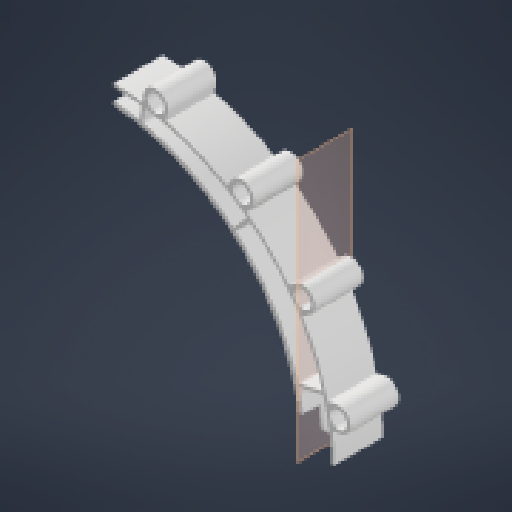
# Autodesk Inventor part: FilterSidewall
Saved by Autodesk Inventor 2026 (Build 300175050, 175E)
## iProperties
Created: 2026-05-05
Part Number: FilterSidewall
Material: Generic
Document SubType Name: Modeling
Designer: sniel
Density: 1 g/cm^3
Appearance: Default
Author: sniel
Autodesk Inventor part; units mm, degrees
ref_plane "YZ Plane" through (0, 0, 0) normal (1, 0, 0) x (0, 1, 0)
ref_plane "XZ Plane" through (0, 0, 0) normal (0, 1, 0) x (-1, 0, 0)
ref_plane "XY Plane" through (0, 0, 0) normal (0, 0, 1) x (1, 0, 0)
sketch "Sketch1" plane through (0, 0, 0) normal (0, 0, 1) x (1, 0, 0)
  circle A0 centre (-26.462672, 2.498755) radius 5.25
  circle A1 centre (-79.388016, -19.42364) radius 5.25
  circle A2 centre (-138.734281, -109.772854) radius 5.25
  circle A3 centre (-116.811886, -56.84751) radius 5.25
  line L0 (-70.374602, -19.468325) -> (-73.075282, -15.258264)
  arc A4 (-73.075282, -15.258264) -> (-85.476982, -23.686741) centre (-79.388065, -19.307803) ccw
  line L1 (-85.476982, -23.686741) -> (-82.556623, -27.747503)
  arc A5 (-82.556623, -27.747503) -> (-108.372236, -53.563116) centre (-0.000049, -136.119689) ccw
  line L2 (-108.372236, -53.563116) -> (-112.432997, -50.642756)
  arc A6 (-112.432997, -50.642756) -> (-120.861475, -63.044456) centre (-116.811935, -56.731673) ccw
  line L3 (-120.861475, -63.044456) -> (-116.651414, -65.745136)
  arc A7 (-116.651414, -65.745136) -> (-132.247344, -103.397042) centre (-0.000049, -136.119689) ccw
  line L4 (-132.247344, -103.397042) -> (-137.133976, -102.329748)
  arc A8 (-137.133976, -102.329748) -> (-139.943468, -117.058908) centre (-138.734331, -109.657017) ccw
  line L5 (-139.943468, -117.058908) -> (-135.00707, -117.865294)
  arc A9 (-135.00707, -117.865294) -> (-136.235526, -136.235526) centre (-0.000049, -136.119689) ccw
  line L6 (-136.235526, -136.235526) -> (-134.235526, -136.235526)
  arc A10 (0, -2) -> (-134.235526, -136.235526) centre (0, -136.235526) ccw
  line L7 (0, -2) -> (0, 0.115837)
  arc A11 (0, 0.115837) -> (-18.254444, -1.112668) centre (-0.000049, -136.119689) ccw
  line L8 (-18.254444, -1.112668) -> (-19.060831, 3.82373)
  arc A12 (-19.060831, 3.82373) -> (-33.78999, 1.014237) centre (-26.462721, 2.614592) ccw
  line L9 (-33.78999, 1.014237) -> (-32.722696, -3.872394)
  arc A13 (-32.722696, -3.872394) -> (-70.374602, -19.468325) centre (-0.000049, -136.119689) ccw
  circle A14 centre (138.734281, -109.772854) radius 5.25
  circle A15 centre (116.811886, -56.84751) radius 5.25
  circle A16 centre (26.462672, 2.498755) radius 5.25
  circle A17 centre (79.388016, -19.42364) radius 5.25
  line L10 (116.651364, -65.745136) -> (120.861425, -63.044456)
  arc A18 (120.861425, -63.044456) -> (112.432948, -50.642756) centre (116.811886, -56.731673) ccw
  line L11 (112.432948, -50.642756) -> (108.372186, -53.563116)
  arc A19 (108.372186, -53.563116) -> (82.556573, -27.747503) centre (0, -136.119689) ccw
  line L12 (82.556573, -27.747503) -> (85.476933, -23.686741)
  arc A20 (85.476933, -23.686741) -> (73.075233, -15.258264) centre (79.388016, -19.307803) ccw
  line L13 (73.075233, -15.258264) -> (70.374553, -19.468325)
  arc A21 (70.374553, -19.468325) -> (32.722647, -3.872394) centre (0, -136.119689) ccw
  line L14 (32.722647, -3.872394) -> (33.789941, 1.014237)
  arc A22 (33.789941, 1.014237) -> (19.060781, 3.82373) centre (26.462672, 2.614592) ccw
  line L15 (19.060781, 3.82373) -> (18.254395, -1.112668)
  arc A23 (18.254395, -1.112668) -> (0, 0.115837) centre (0, -136.119689) ccw
  line L16 (0, 0.115837) -> (0, -2)
  arc A24 (134.235526, -136.235526) -> (0, -2) centre (0, -136.235526) ccw
  line L17 (134.235526, -136.235526) -> (136.235477, -136.235526)
  arc A25 (136.235477, -136.235526) -> (135.007021, -117.865294) centre (0, -136.119689) ccw
  line L18 (135.007021, -117.865294) -> (139.943419, -117.058908)
  arc A26 (139.943419, -117.058908) -> (137.133926, -102.329748) centre (138.734281, -109.657017) ccw
  line L19 (137.133926, -102.329748) -> (132.247295, -103.397042)
  arc A27 (132.247295, -103.397042) -> (116.651364, -65.745136) centre (0, -136.119689) ccw
  arc A28 (132.235526, -136.235526) -> (0, -4) centre (0, -136.235526) ccw
  line L20 (0, -4) -> (0, -31)
  arc A29 (105.235526, -136.235526) -> (0, -31) centre (0, -136.235526) ccw
  line L21 (105.235526, -136.235526) -> (132.235526, -136.235526)
  arc A30 (0, -4) -> (-132.235526, -136.235526) centre (0, -136.235526) ccw
  line L22 (-132.235526, -136.235526) -> (-105.235526, -136.235526)
  arc A31 (0, -31) -> (-105.235526, -136.235526) centre (0, -136.235526) ccw
  line L23 (0, -31) -> (0, -4)
  line L24 (105.235526, -136.235526) -> (115.235526, -136.235526)
  line L25 (132.235526, -136.235526) -> (118.235526, -136.235526)
  arc A32 (115.235526, -136.235526) -> (-134.235526, -136.235526) centre (-9.5, -136.235526) ccw
  arc A33 (118.235526, -136.235526) -> (-136.235526, -136.235526) centre (-9, -136.127341) ccw
  line L26 (17.913319, -3.200608) -> (16.630384, -11.5)
  line L27 (16.630384, -11.5) -> (18.586158, -11.918265)
  line L28 (18.586158, -11.918265) -> (19.890284, -3.481795)
  line L29 (73.979575, -39.673825) -> (82.556573, -30.38852)
  line L30 (73.979575, -39.673825) -> (75.485418, -40.990046)
  line L31 (75.485418, -40.990046) -> (84.128311, -31.633405)
  line L32 (113.810426, -102.863395) -> (114.318109, -104.797887)
  line L33 (114.318109, -104.797887) -> (129.649883, -101.449261)
  line L34 (113.810426, -102.863395) -> (129.11688, -99.520299)
  point P0 (-105.180629, -52.831618)
  dimension "d17" = 10
  dimension "d18" = 14
  dimension "d28" = 2
  dimension "d29" = 2
  dimension "d31" = 2
  constraints: 62 end point, 56 point on circle, 30 centre point, 3 parallel, 2 point on line, 2 tangent
  measures "d17" distance of L21.start L24.end
  measures "d18" distance of L21.end L25.end
  measures "d28" distance of L26.end L27.end
  measures "d29" distance of L29.start L30.end
  measures "d31" distance of L32.start L32.end
extrude "Extrusion1" add sketch "Sketch1" along normal blind 30 contours A2 A33 A9 L5 A8 L4 A7 L3 A6 L2 A5 L1 A4 L0 A13 L9 A12 L8 A11 L7 A10 | A2 A33 A10 L6 | A33 A30 A32 A10 | L7 A23 L15 A22 L14 A21 L13 A20 L12 A19 L11 A18 L10 A27 L19 A26 L18 A25 L17 A24 | A33 L20 A32 A30 | A24 L28 A28 L26 | A33 L27 L30 L32 L21 A32 L20 | A28 L28 A33 L26 | A33 L27 | A24 L31 A28 L29 | A28 L31 A33 L29 | A33 L30 | L32 A33 | A33 L34 A28 L33 | A24 L33 A28 L34
ref_plane "Work Plane1" through (115.235526, -136.235526, 0) normal (1, 0, 0) x (0, 0, 1)
sketch "Sketch2" plane through (115.235526, -136.235526, 0) normal (1, 0, 0) x (0, 0, 1)
  line L0 (0, 0) -> (30, 0)
  line L1 (30, 0) -> (30, -124.735526)
  line L2 (0, 0) -> (0, -124.735526)
  line L3 (0, 0) -> (22, 0)
  line L4 (11, 0) -> (11, -7.5)
  circle A0 centre (11, -7.5) radius 7.5
  line L5 (18.5, -7.5) -> (18.5, -17.5)
  line L6 (3.5, -7.5) -> (3.5, -17.5)
  line L7 (3.5, -17.5) -> (0, -17.5)
  line L8 (18.5, -17.5) -> (30, -17.5)
  point P0 (0, -136.235526)
  point P1 (11, 0)
  dimension "d21" = 22
  dimension "d22" = 7.5
  dimension "d23" = 10
  constraints: 12 end point, 4 point on line, 3 point on circle, 3 vertical, 1 centre point, 1 coincident, 1 midpoint, 1 perpendicular, 1 tangent
  measures "d21" distance of L0.start L3.end
  measures "d22" distance of L4.start L4.end
  measures "d23" distance of L5.start L5.end
extrude "Extrusion2" cut sketch "Sketch2" along normal mid plane 13.75 contours L0 A0 L6 L7 L2 | L0 L1 L8 L5 A0
sketch "Sketch3" plane through (0, 0, 30) normal (0, 0, 1) x (1, 0, 0)
  line L0 (114.001828, -118.735526) -> (117.041325, -118.735526)
  arc A0 (117.041325, -118.735526) -> (-105.180629, -52.831618) centre (-9, -136.127341) ccw
  arc A1 (134.235526, -136.235526) -> (-105.180629, -52.831618) centre (0, -136.235526) ccw
  line L1 (134.235526, -136.235526) -> (136.235477, -136.235526)
  arc A2 (136.235477, -136.235526) -> (135.007021, -117.865294) centre (0, -136.119689) ccw
  line L2 (135.007021, -117.865294) -> (139.943419, -117.058908)
  arc A3 (139.943419, -117.058908) -> (137.133926, -102.329748) centre (138.734281, -109.657017) ccw
  line L3 (137.133926, -102.329748) -> (132.247295, -103.397042)
  arc A4 (132.247295, -103.397042) -> (116.651364, -65.745136) centre (0, -136.119689) ccw
  line L4 (116.651364, -65.745136) -> (120.861425, -63.044456)
  arc A5 (120.861425, -63.044456) -> (112.432948, -50.642756) centre (116.811886, -56.731673) ccw
  line L5 (112.432948, -50.642756) -> (108.372186, -53.563116)
  arc A6 (108.372186, -53.563116) -> (82.556573, -27.747503) centre (0, -136.119689) ccw
  line L6 (82.556573, -27.747503) -> (85.476933, -23.686741)
  arc A7 (85.476933, -23.686741) -> (73.075233, -15.258264) centre (79.388016, -19.307803) ccw
  line L7 (73.075233, -15.258264) -> (70.374553, -19.468325)
  arc A8 (70.374553, -19.468325) -> (32.722647, -3.872394) centre (0, -136.119689) ccw
  line L8 (32.722647, -3.872394) -> (33.789941, 1.014237)
  arc A9 (33.789941, 1.014237) -> (19.060781, 3.82373) centre (26.462672, 2.614592) ccw
  line L9 (19.060781, 3.82373) -> (18.254395, -1.112668)
  arc A10 (18.254395, -1.112668) -> (-18.254444, -1.112668) centre (-0.000025, -136.120055) ccw
  line L10 (-18.254444, -1.112668) -> (-19.060831, 3.82373)
  arc A11 (-19.060831, 3.82373) -> (-33.78999, 1.014237) centre (-26.462721, 2.614592) ccw
  line L11 (-33.78999, 1.014237) -> (-32.722696, -3.872394)
  arc A12 (-32.722696, -3.872394) -> (-70.374602, -19.468325) centre (-0.000049, -136.119689) ccw
  line L12 (-70.374602, -19.468325) -> (-73.075282, -15.258264)
  arc A13 (-73.075282, -15.258264) -> (-85.476982, -23.686741) centre (-79.388065, -19.307803) ccw
  line L13 (-85.476982, -23.686741) -> (-82.556623, -27.747503)
  arc A14 (-82.556623, -27.747503) -> (-108.372236, -53.563116) centre (-0.000049, -136.119689) ccw
  line L14 (-108.372236, -53.563116) -> (-112.432997, -50.642756)
  arc A15 (-112.432997, -50.642756) -> (-120.861475, -63.044456) centre (-116.811935, -56.731673) ccw
  line L15 (-120.861475, -63.044456) -> (-116.651414, -65.745136)
  arc A16 (-116.651414, -65.745136) -> (-132.247344, -103.397042) centre (-0.000049, -136.119689) ccw
  line L16 (-132.247344, -103.397042) -> (-137.133976, -102.329748)
  arc A17 (-137.133976, -102.329748) -> (-139.943468, -117.058908) centre (-138.734331, -109.657017) ccw
  line L17 (-139.943468, -117.058908) -> (-135.00707, -117.865294)
  arc A18 (-135.00707, -117.865294) -> (-136.235526, -136.235526) centre (-0.000049, -136.119689) ccw
  line L18 (-136.235526, -136.235526) -> (-134.235526, -136.235526)
  arc A19 (114.001828, -118.735526) -> (-134.235526, -136.235526) centre (-9.5, -136.235526) ccw
  circle A20 centre (138.734281, -109.772854) radius 5.25
  circle A21 centre (116.811886, -56.84751) radius 5.25
  circle A22 centre (26.462672, 2.498755) radius 5.25
  circle A23 centre (79.388016, -19.42364) radius 5.25
  circle A24 centre (-138.734281, -109.772854) radius 5.25
  circle A25 centre (-116.811886, -56.84751) radius 5.25
  circle A26 centre (-79.388016, -19.42364) radius 5.25
  circle A27 centre (-26.462672, 2.498755) radius 5.25
  line L19 (-0.000025, 0.115837) -> (-0.000025, -11.86229)
  point P0 (-0.000025, -9.210474)
  point P1 (-0.000025, -2)
  constraints: 56 centre point, 42 point on circle, 40 end point, 1 vertical
extrude "Extrusion3" cut sketch "Sketch3" against normal blind 31 contours A19 L18 A18 L17 A17 L16 A16 L15 A15 L14 A14 L13 A13 L12 A12 L11 A11 L10 A10 L19 A1 A0
fillet "Fillet1" radius 1 30 edges at (0, 0.1158, 15) (0, -2, 15) (0, -9.2105, 15) (0, -11.8623, 15) (17.9133, -3.2006, 15) (19.8903, -3.4818, 15) (16.6304, -11.5, 15) (18.5862, -11.9183, 15) (73.9796, -39.6738, 15) (75.4854, -40.99, 15) (84.1283, -31.6334, 15) (82.5566, -30.3885, 15) (117.0413, -118.7355, 24.25) (114.0018, -118.7355, 24.25) (115.2229, -134.4612, 15.8443) (115.2231, -134.4758, 6.173) (114.6066, -123.7254, 3.5) (114.6066, -123.7254, 18.5) (118.2247, -134.4613, 15.8441) (118.2249, -134.4759, 6.1732) (117.6298, -123.7259, 3.5) (117.6298, -123.7259, 18.5) (114.0018, -118.7355, 1.75) (117.0413, -118.7355, 1.75) (129.6499, -101.4493, 15) (114.3181, -104.7979, 15) (113.8104, -102.8634, 15) (129.1169, -99.5203, 15) (134.2355, -136.2355, 15) (136.2355, -136.2355, 15)
body "Solid1"
